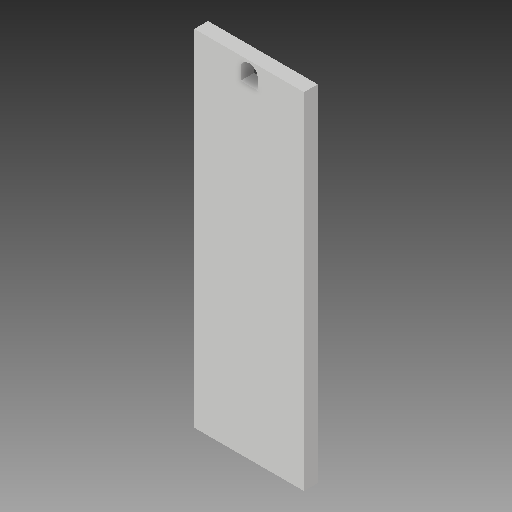
# Autodesk Inventor part: base_fixaxao_cabeca_supeior
Saved by Autodesk Inventor 2018 (Build 220112000, 112)
## iProperties
Created: 2018-07-04
Part Number: base_fixaxao_cabeca_supeior
Material: Genérico
Document SubType Name: Modeling
Designer: Usuario
Density: 1 g/cm^3
Appearance: Padrão
Mass: 172.696 g
Surface Area: 427.394 cm^2
Volume: 172.696 cm^3
Author: Usuario
Autodesk Inventor part; units mm, degrees
ref_plane "YZ Plane" through (0, 0, 0) normal (1, 0, 0) x (0, 1, 0)
ref_plane "XZ Plane" through (0, 0, 0) normal (0, 1, 0) x (-1, 0, 0)
ref_plane "XY Plane" through (0, 0, 0) normal (0, 0, 1) x (1, 0, 0)
sketch "Esboço2" plane through (0, 0, 0) normal (0, 0, 1) x (1, 0, 0)
  line L0 (-38.1, 120) -> (38.1, 120)
  line L1 (38.1, 120) -> (38.1, -120)
  line L2 (38.1, -120) -> (-38.1, -120)
  line L3 (-38.1, -120) -> (-38.1, 120)
  line L4 (-38.1, 120) -> (38.1, -120) construction
  line L5 (38.1, 120) -> (-38.1, -120) construction
  point P0 (0, 0)
  dimension "d6" = 76.2
  dimension "d7" = 240
  constraints: 12 end point, 2 midpoint, 2 parallel, 1 horizontal, 1 perpendicular
  measures "d6" distance of L1.end L2.end
  measures "d7" distance of L0.end L1.end
extrude "Extrusão2" add sketch "Esboço2" against normal blind 9.52
sketch "Esboço3" plane through (0, 0, -9.52) normal (0, 0, -1) x (-1, 0, 0)
  line L0 (0, 120) -> (0, 104.8191) construction
  line L1 (0, 104.8191) -> (-38.1, 104.8191) construction
  line L2 (-38.1, 120) -> (-38.1, -120) projected
  line L3 (0, 104.8191) -> (38.1, 104.8191) construction
  line L4 (38.1, -120) -> (38.1, 120) projected
  arc A0 (6, 112.4095) -> (-6, 112.4095) centre (0, 112.4095) ccw
  line L5 (-6, 112.4095) -> (-6, 104.8191)
  line L6 (6, 104.8191) -> (6, 112.4095)
  line L7 (-6, 104.8191) -> (6, 104.8191)
  point P0 (0, 0)
  dimension "d10" = 12
  constraints: 12 end point, 5 point on line, 2 perpendicular, 2 point on circle, 1 centre point, 1 collinear, 1 midpoint, 1 parallel, 1 tangent, 1 vertical
  measures "d10" diameter of A0
extrude "Extrusão3" cut sketch "Esboço3" against normal through all
